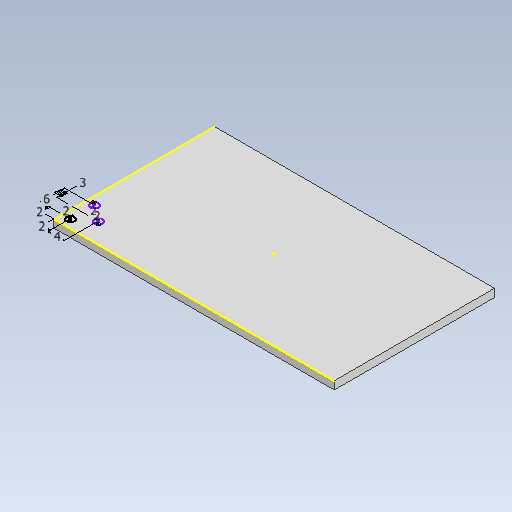
# Autodesk Inventor part: base_soft
Saved by Autodesk Inventor 2020 (Build 240168000, 168)
## iProperties
Created: 2020-01-22
Part Number: base_soft
Material: Generic
Document SubType Name: Modeling
Designer: sl65b
Density: 1 g/cm^3
Appearance: Default
Author: sl65b
Autodesk Inventor part; units mm, degrees
ref_plane "YZ Plane" through (0, 0, 0) normal (1, 0, 0) x (0, 1, 0)
ref_plane "XZ Plane" through (0, 0, 0) normal (0, 1, 0) x (-1, 0, 0)
ref_plane "XY Plane" through (0, 0, 0) normal (0, 0, 1) x (1, 0, 0)
sketch "Sketch1" plane through (0, 0, 0) normal (0, 1, 0) x (-1, 0, 0)
  line L0 (-35, -20) -> (35, -20)
  line L1 (35, -20) -> (35, 20)
  line L2 (35, 20) -> (-35, 20)
  line L3 (-35, 20) -> (-35, -20)
  line L4 (-35, -20) -> (35, 20) construction
  line L5 (35, -20) -> (-35, 20) construction
  point P0 (0, 0)
  dimension "d0" = 70
  dimension "d1" = 40
  constraints: 12 end point, 2 midpoint, 2 parallel, 1 horizontal, 1 perpendicular
  measures "d0" distance of L2.end L1.end
  measures "d1" distance of L0.end L1.end
extrude "Extrusion1" add sketch "Sketch1" along normal blind 2
sketch "Sketch2" plane through (0, 2, 0) normal (0, 1, 0) x (1, 0, 0)
  circle A0 centre (-33, -18) radius 1
  line L0 (-35, -20) -> (35, -20) projected
  line L1 (-35, 20) -> (-35, -20) projected
  circle A1 centre (-33, -12) radius 1
  circle A2 centre (-29, -15) radius 1
  point P0 (0, 0)
  dimension "d4" = 2
  dimension "d5" = 2
  dimension "d6" = 2
  dimension "d7" = 2
  dimension "d8" = 6
  dimension "d9" = 2
  dimension "d11" = 4
  dimension "d12" = 3
  constraints: 3 centre point
  measures "d4" diameter of A0
  measures "d5" distance from line of L0 A0.centre
  measures "d6" distance from line of L1 A0.centre
  measures "d7" diameter of A1
  measures "d8" distance of A0.centre A1.centre
  measures "d9" diameter of A2
  measures "d11" horizontal distance of A0.centre A2.centre
  measures "d12" vertical distance of A1.centre A2.centre
body "Solid1"
